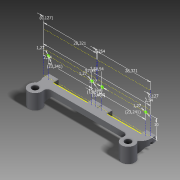
# Autodesk Inventor part: HDMIPluginModuleHolder02
Saved by Autodesk Inventor 2015 (Build 190159000, 159)
## iProperties
Created: 2015-10-14
Part Number: HDMIPluginModuleHolder02
Material: Generic
Document SubType Name: Modeling
Designer: -
Density: 1 g/cm^3
Appearance: Default
Author: -
Autodesk Inventor part; units mm, degrees
ref_plane "YZ Plane" through (0, 0, 0) normal (1, 0, 0) x (0, 1, 0)
ref_plane "XZ Plane" through (0, 0, 0) normal (0, 1, 0) x (-1, 0, 0)
ref_plane "XY Plane" through (0, 0, 0) normal (0, 0, 1) x (1, 0, 0)
sketch "Sketch1" plane through (0, 0, 0) normal (0, 1, 0) x (-1, 0, 0)
  circle A0 centre (0, 0) radius 1.65
  line L0 (0, 0) -> (22.867074, 0) construction
  circle A1 centre (-49.53, 0) radius 1.65
  circle A2 centre (-49.53, 0) radius 3.5
  line L1 (-24.765, 0) -> (-24.765, 33.489729) construction
  line L2 (0, 0) -> (0, -6.321967) construction
  line L3 (-49.53, 0) -> (-44.53, 0) construction
  circle A3 centre (0, 0) radius 3.5
  dimension "d0" = 3.3
  dimension "d2" = 49.53
  dimension "d3" = 3.3
  dimension "d4" = 7
  dimension "d11" = 7
  constraints: 8 end point, 4 centre point, 3 coincident, 2 horizontal, 2 vertical, 1 point on line
  measures "d0" diameter of A0
  measures "d2" distance of L0.start A1.centre
  measures "d3" diameter of A1
  measures "d4" diameter of A2
  measures "d11" diameter of A3
extrude "Extrusion1" add sketch "Sketch1" along normal blind 3
sketch "Sketch2" plane through (49.53, 0, 0) normal (0, -1, 0) x (1, 0, 0)
  line L0 (2, -2.2) -> (2, -5.2)
  line L1 (0, -7.2) -> (-49.53, -7.2)
  line L2 (-51.53, -5.2) -> (-51.53, -2.2)
  line L3 (-47.53, -2.2) -> (-47.53, -2.2)
  line L4 (-46.53, -3.2) -> (-3, -3.2)
  line L5 (-2, -2.2) -> (-2, -2.2)
  line L6 (0, 0) -> (0, -7.711546) construction
  line L7 (2, -2.2) -> (-2, -2.2)
  line L8 (-49.53, 0) -> (-49.53, -7.241497) construction
  line L9 (-47.53, -2.2) -> (-51.53, -2.2)
  arc A0 (-47.53, -2.2) -> (-46.53, -3.2) centre (-46.53, -2.2) ccw
  arc A1 (-3, -3.2) -> (-2, -2.2) centre (-3, -2.2) ccw
  arc A2 (-51.53, -5.2) -> (-49.53, -7.2) centre (-49.53, -5.2) ccw
  arc A3 (0, -7.2) -> (2, -5.2) centre (0, -5.2) ccw
  point P0 (2, -7.2)
  point P1 (0, -2.2)
  point P2 (-49.53, -2.2)
  dimension "d14" = 5
  dimension "d15" = 2.2
  dimension "d16" = 4
  dimension "d17" = 4
  dimension "d18" = 2.2
  dimension "d19" = 1
  dimension "d20" = 2
  constraints: 20 end point, 8 point on circle, 8 tangent, 4 centre point, 4 perpendicular, 4 point on line, 3 vertical, 2 equal radius, 2 horizontal, 2 midpoint, 2 other
  measures "d14" distance of L0.start point (2, -7.2)
  measures "d15" distance from line of L6.start L7
  measures "d16" distance between parallel lines of L0 L5
  measures "d17" distance between parallel lines of L4 L1
  measures "d18" distance from line of L8.start L9
  measures "d19" radius of A0
  measures "d20" radius of A2
extrude "Extrusion2" add sketch "Sketch2" against normal blind 3
sketch "Sketch3" plane through (49.53, 0, -7.2) normal (0, 0, -1) x (-1, 0, 0)
  arc A0 (20.526777, 0.5715) -> (21.669777, 0.5715) centre (21.098277, 0.5715) ccw
  line L0 (49.53, 0) -> (0, 0) construction
  line L1 (0, 3) -> (49.53, 3)
  line L2 (-2, 0) -> (-2, 3)
  line L3 (21.669777, 0.5715) -> (21.669777, 1.2065)
  line L4 (21.669777, 1.2065) -> (23.669777, 1.2065)
  line L5 (23.669777, 1.2065) -> (23.669777, 3)
  line L6 (20.526777, 0.5715) -> (20.526777, 1.2065)
  line L7 (20.526777, 1.2065) -> (18.526777, 1.2065)
  line L8 (18.526777, 1.2065) -> (18.526777, 3)
  line L9 (21.098277, 0.5715) -> (22.273198, 0.5715) construction
  line L10 (23.669777, 3) -> (18.526777, 3)
  point P0 (49.53, 0)
  point P1 (46.53, 3)
  point P2 (3, 3)
  dimension "d23" = 1.143
  dimension "d26" = 23.09828
  dimension "d27" = 2
  dimension "d28" = 2
  dimension "d29" = 0.635
  dimension "d30" = 0.635
  dimension "d31" = 2.4285
  constraints: 16 end point, 3 perpendicular, 2 collinear, 2 horizontal, 2 point on circle, 2 point on line, 2 vertical, 1 centre point, 1 coincident, 1 tangent
  measures "d23" diameter of A0
  measures "d26" distance from line of A0.centre L2
  measures "d27" distance of L3.end L4.end
  measures "d28" distance of L6.end L7.end
  measures "d29" distance of L6.start L6.end
  measures "d30" distance of L3.start L3.end
  measures "d31" distance from line of L9.start L10
extrude "Extrusion3" add sketch "Sketch3" along normal blind 3
pattern_linear "Rectangular Pattern1" count 2 spacing 23.241 along (1, 0, 0) of "Extrusion3"
sketch "Sketch4" plane through (49.101223, 3, -7.2) normal (0, 1, 0) x (1, 0, 0)
  arc A0 (0, -5.143) -> (5.143, 0) centre (0, 0) ccw
  line L0 (5.143, 0) -> (0, 0)
  line L1 (0, 0) -> (0, -5.143)
  point P0 (-49.101223, -7.2)
  constraints: 4 end point, 2 point on circle, 1 centre point, 1 horizontal, 1 perpendicular
extrude "Extrusion4" add sketch "Sketch4" against normal blind 3
pattern_linear "Rectangular Pattern2" count 2 spacing 5.334 along (-1, 0, 0) of "Extrusion3"
pattern_linear "Rectangular Pattern3" count 2 spacing 28.575 along (-1, 0, 0) of "Extrusion3"
sketch "Sketch6" plane through (-2.714777, 3, -7.2) normal (0, 1, 0) x (1, 0, 0)
  arc A0 (0, 0) -> (3.143, -3.143) centre (3.143, 0) ccw
  line L0 (3.143, -3.143) -> (3.143, 0)
  line L1 (3.143, 0) -> (0, 0)
  point P0 (2.714777, -7.2)
  constraints: 4 end point, 2 point on circle, 1 centre point, 1 perpendicular, 1 vertical
extrude "Extrusion5" add sketch "Sketch6" against normal blind 3
sketch "Sketch7" plane through (54.244223, 3, -10.2) normal (0, 0, -1) x (-1, 0, 0)
  line L0 (3.143, -2.4285) -> (3.143, -1.7935) construction
  line L1 (3.143, -1.7935) -> (5.143, -1.7935) construction
  line L2 (5.143, -1.7935) -> (5.143, 0) construction
  line L3 (5.143, 0) -> (0, 0) construction
  line L4 (0, 0) -> (0, -1.7935) construction
  line L5 (0, -1.7935) -> (2, -1.7935) construction
  line L6 (2, -1.7935) -> (2, -2.4285) construction
  arc A0 (2, -2.4285) -> (3.143, -2.4285) centre (2.5715, -2.4285) ccw construction
  line L7 (0, -1.7935) -> (0, 0)
  line L8 (0, 0) -> (5.143, 0)
  line L9 (5.143, 0) -> (5.143, -1.7935)
  arc A1 (0, -1.7935) -> (5.143, -1.7935) centre (2.5715, -1.7935) ccw
  line L10 (5.143, -1.7935) -> (0, -1.7935) construction
  line L11 (5.143, -1.7935) -> (5.143, 0) construction
  point P0 (54.244223, -3)
  constraints: 8 end point, 3 perpendicular, 2 point on circle, 1 centre point, 1 coincident, 1 midpoint, 1 vertical
extrude "Extrusion6" add sketch "Sketch7" against normal blind 1.2
pattern_linear "Rectangular Pattern4" count 2 spacing 23.241 along (-1, 0, 0) of "Extrusion6"
pattern_linear "Rectangular Pattern5" count 2 spacing 28.575 along (-1, 0, 0) of "Extrusion6"
pattern_linear "Rectangular Pattern6" count 2 spacing 51.816 along (-1, 0, 0) of "Extrusion6"
sketch "Sketch8" plane through (49.53, 0, -7.2) normal (0, 0, -1) x (-1, 0, 0)
  line L0 (-4.809723, 14.023831) -> (52.340277, 14.023831) construction
  line L1 (52.340277, 14.023831) -> (52.340277, 4.023831) construction
  line L2 (52.340277, 4.023831) -> (-4.809723, 4.023831) construction
  line L3 (-4.809723, 4.023831) -> (-4.809723, 14.023831) construction
  line L4 (-4.682723, 25.302039) -> (23.638277, 25.302039) construction
  line L5 (23.638277, 25.302039) -> (23.638277, 16.254183) construction
  line L6 (23.638277, 16.254183) -> (-4.682723, 16.254183) construction
  line L7 (-4.682723, 16.254183) -> (-4.682723, 25.302039) construction
  line L8 (52.213277, 25.302039) -> (23.892277, 25.302039) construction
  line L9 (23.892277, 25.302039) -> (23.892277, 16.254183) construction
  line L10 (23.892277, 16.254183) -> (52.213277, 16.254183) construction
  line L11 (52.213277, 16.254183) -> (52.213277, 25.302039) construction
  circle A0 centre (-2.142723, 14.023831) radius 0.635
  circle A1 centre (21.098277, 14.023831) radius 0.635
  circle A2 centre (26.432277, 14.023831) radius 0.635
  circle A3 centre (49.673277, 14.023831) radius 0.635
  arc A4 (-2.714223, 0.5715) -> (-1.571223, 0.5715) centre (-2.142723, 0.5715) ccw
  line L12 (-2.142723, 0.5715) -> (-2.142723, 10.619847) construction
  arc A5 (20.526777, 0.5715) -> (21.669777, 0.5715) centre (21.098277, 0.5715) ccw construction
  arc A6 (25.860777, 0.5715) -> (27.003777, 0.5715) centre (26.432277, 0.5715) ccw construction
  arc A7 (49.101777, 0.5715) -> (50.244777, 0.5715) centre (49.673277, 0.5) ccw construction
  line L13 (21.098277, 0.5715) -> (21.098277, 9.023831) construction
  line L14 (26.432277, 0.5715) -> (26.432277, 8.168185) construction
  line L15 (49.673277, 0.5) -> (49.673277, 8.952331) construction
  line L16 (23.860777, 1.2065) -> (23.860777, 3) construction
  line L17 (23.669777, 3) -> (23.860777, 3) construction
  line L18 (23.669777, 3) -> (23.669777, 1.2065) construction
  line L19 (23.669777, 1.2065) -> (21.669777, 1.2065) construction
  line L20 (21.669777, 1.2065) -> (21.669777, 0.5715) construction
  arc A8 (21.098277, 0) -> (21.669777, 0.5715) centre (21.098277, 0.5715) ccw construction
  line L21 (20.526777, 0.5715) -> (20.526777, 1.2065) construction
  line L22 (20.526777, 1.2065) -> (18.526777, 1.2065) construction
  line L23 (18.526777, 1.2065) -> (18.526777, 3) construction
  line L24 (29.003777, 3) -> (29.003777, 1.2065) construction
  line L25 (29.003777, 1.2065) -> (27.003777, 1.2065) construction
  line L26 (27.003777, 1.2065) -> (27.003777, 0.5715) construction
  arc A9 (26.432277, 0) -> (27.003777, 0.5715) centre (26.432277, 0.5715) ccw construction
  line L27 (25.860777, 0.5715) -> (25.860777, 1.2065) construction
  line L28 (25.860777, 1.2065) -> (23.860777, 1.2065) construction
  line L29 (49.53, 0) -> (0, 0) construction
  line L30 (24.765, 0) -> (24.765, 9.663085) construction
  line L31 (47.101777, 1.2065) -> (47.101777, 3)
  line L32 (49.101777, 0.5715) -> (49.101777, 1.2065)
  line L33 (49.101777, 1.2065) -> (47.101777, 1.2065)
  line L34 (0.428777, 1.2065) -> (-1.571223, 1.2065)
  line L35 (-1.571223, 1.2065) -> (-1.571223, 0.5715)
  line L36 (0.428777, 3) -> (18.526777, 3)
  line L37 (0.428777, 3) -> (0.428777, 1.2065)
  arc A10 (-2.142723, 0) -> (-1.571223, 0.5715) centre (-2.142723, 0.5715) ccw
  line L38 (29.003777, 3) -> (47.101777, 3)
  line L39 (21.098277, 0) -> (-2.142723, 0)
  line L40 (26.432277, 0) -> (21.098277, 0)
  arc A11 (20.526777, 0.5715) -> (21.098277, 0) centre (21.098277, 0.5715) ccw
  arc A12 (25.860777, 0.5715) -> (26.432277, 0) centre (26.432277, 0.5715) ccw
  line L41 (49.673277, 0) -> (26.432277, 0)
  arc A13 (49.101777, 0.5715) -> (49.673277, 0) centre (49.673277, 0.5715) ccw
  point P0 (49.53, 0)
  point P1 (49.396488, 0)
  point P2 (49.53, 0.018251)
  dimension "d57" = 57.15
  dimension "d58" = 10
  dimension "d59" = 28.321
  dimension "d60" = 0.127
  dimension "d61" = 28.321
  dimension "d62" = 0.254
  dimension "d63" = 0.127
  dimension "d64" = 1.27
  dimension "d65" = 2.54
  dimension "d66" = 1.27
  dimension "d67" = 2.54
  dimension "d68" = 1.27
  dimension "d69" = 1.27
  dimension "d70" = 2.54
  dimension "d71" = 2.54
  dimension "d72" = 23.241
  dimension "d73" = 5.334
  dimension "d74" = 23.241
  dimension "d75" = 1.66728
  dimension "d76" = 3.66672
  constraints: 34 end point, 6 parallel, 5 point on line, 5 vertical, 4 centre point, 3 horizontal, 3 perpendicular, 1 collinear, 1 midpoint, 1 other
  measures "d57" distance of L0.start L0.end
  measures "d58" distance of L2.end L0.start
  measures "d59" distance of L4.start L4.end
  measures "d60" distance between parallel lines of L3 L7
  measures "d61" distance of L8.start L8.end
  measures "d62" distance between parallel lines of L5 L9
  measures "d63" distance between parallel lines of L11 L1
  measures "d64" diameter of A0
  measures "d65" distance from line of L7 A0.centre
  measures "d66" diameter of A1
  measures "d67" distance from line of A1.centre L5
  measures "d68" diameter of A3
  measures "d69" diameter of A2
  measures "d70" distance from line of L9 A2.centre
  measures "d71" distance from line of L11 A3.centre
  measures "d72" distance of A0.centre A1.centre
  measures "d73" distance of A1.centre A2.centre
  measures "d74" distance of A3.centre A2.centre
  measures "d75" distance from line of L30 A2.centre
  measures "d76" distance from line of A1.centre L30
sketch "Sketch9" plane through (0, 0, 0) normal (0, -1, 0) x (1, 0, 0)
  circle A0 centre (0, 0) radius 1.65
  circle A1 centre (49.53, 0) radius 1.65
  circle A2 centre (49.53, 0) radius 3.5
  arc A3 (2.164913, -2.750118) -> (-2, -2.872281) centre (0, 0) ccw
  circle A4 centre (0, 0) radius 3.5
  constraints: 2 centre point, 2 coincident
extrude "Extrusion7" add sketch "Sketch9" along normal blind 5
chamfer "Chamfer1" distance 3 angle 45 1 edges at (49.5259, 0, -3.5)
chamfer "Chamfer2" distance 3 angle 45 1 edges at (0.1026, 0, -3.4985)
fillet "Fillet1" radius 2 3 edges at (47.3651, 0, -2.7501) (2.1649, 1.5, -2.7501) (2.1649, -1.5, -2.7501)
body "Solid1"
